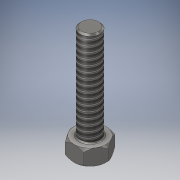
# Autodesk Inventor part: porca m6
Saved by Autodesk Inventor 2019.4 (Build 234330000, 330)
## iProperties
Created: 2020-08-26
Part Number: porca m6
Material: Aço inoxidável
Document SubType Name: Modeling
Designer: Lattes
Density: 8 g/cm^3
Appearance: Semipolido
Author: Lattes
Autodesk Inventor part; units mm, degrees
ref_plane "YZ Plane" through (0, 0, 0) normal (1, 0, 0) x (0, 1, 0)
ref_plane "XZ Plane" through (0, 0, 0) normal (0, 1, 0) x (-1, 0, 0)
ref_plane "XY Plane" through (0, 0, 0) normal (0, 0, 1) x (1, 0, 0)
sketch "Esboço1" plane through (0, 0, 0) normal (0, 1, 0) x (-1, 0, 0)
  circle A0 centre (0, 0) radius 3
  line L0 (-2.8868, -5) -> (-5.7735, 0)
  line L1 (-5.7735, 0) -> (-2.8868, 5)
  line L2 (-2.8868, 5) -> (2.8868, 5)
  line L3 (2.8868, 5) -> (5.7735, 0)
  line L4 (5.7735, 0) -> (2.8868, -5)
  line L5 (2.8868, -5) -> (-2.8868, -5)
  dimension "d0" = 6
  constraints: 12 end point, 2 coincident, 1 centre point, 13 other
  measures "d0" diameter of A0
extrude "Extrusão1" add sketch "Esboço1" along normal blind 5
sketch "Esboço2" plane through (0, 0, 0) normal (1, 0, 0) x (0, 1, 0)
  point P0 (0, 0)
chamfer "Chanfro1" distance 0.5 angle 45 2 edges at (3, 0, 0) (3, 5, 0)
sketch "Esboço5" plane through (0, 0, 0) normal (0, -1, 0) x (1, 0, 0)
  circle A0 centre (0, 0) radius 5
  constraints: 1 centre point, 1 coincident
extrude "Extrusão2" cut sketch "Esboço5" against normal through all draft 45 keep common part
sketch "Esboço6" plane through (0, 5, 0) normal (0, 1, 0) x (1, 0, 0)
  circle A0 centre (0, 0) radius 5
  constraints: 1 centre point, 1 coincident
extrude "Extrusão3" cut sketch "Esboço6" against normal through all draft 45 keep common part
sketch "Esboço7" plane through (0, 5, 0) normal (0, 1, 0) x (1, 0, 0)
  circle A0 centre (0, 0) radius 3.5
  constraints: 1 centre point, 1 coincident
extrude "Extrusão4" add sketch "Esboço7" against normal blind 5
sketch "Esboço8" plane through (0, 5, 0) normal (0, 1, 0) x (1, 0, 0)
  circle A0 centre (0, 0) radius 3.175
  dimension "d16" = 6.35
  constraints: 1 centre point, 1 coincident
  measures "d16" diameter of A0
extrude "Extrusão5" add sketch "Esboço8" along normal blind 30
fillet "Arredondamento2" radius 0.4 1 edges at (-3.175, 5, 0)
chamfer "Chanfro3" distance 0.5 angle 45 1 edges at (-3.175, 35, 0)
thread "Rosca3" size "1/4-14" class "2B" standard "Inch Tapping Threads" full length
